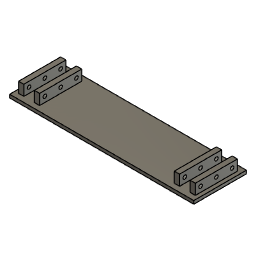
Base v1 (Autodesk Fusion 360 design; units mm, degrees)
Autodesk Fusion 360 part; units mm, degrees
sketch "Sketch1" plane through (0, 0, 0) normal (0, 1, 0) x (1, 0, 0)
  line L0 (-25, 5) -> (150, 5)
  line L1 (150, 5) -> (150, -45)
  line L2 (150, -45) -> (-25, -45)
  line L3 (-25, -45) -> (-25, 5)
  dimension "d1" = 50
  dimension "d2" = 175
  constraint horizontal L0
  constraint vertical L1
  constraint horizontal L2
  constraint vertical L3
  measures "d1" distance of L0.start L2.end
  measures "d2" distance of L0.start L0.end
extrude "Extrude1" add sketch "Sketch1" along normal blind 3
sketch "Sketch2" plane through (0, 3, 0) normal (0, 1, 0) x (-1, 0, 0)
  line L0 (25, 45) -> (-150, 45)
  line L1 (-150, 45) -> (-150, -5)
  line L2 (-150, -5) -> (25, -5)
  line L3 (25, -5) -> (25, 45)
  line L4 (21.5, 0) -> (16.5, 0)
  line L5 (16.5, 0) -> (16.5, 40)
  line L6 (16.5, 40) -> (21.5, 40)
  line L7 (21.5, 40) -> (21.5, 0)
  line L8 (-141.5, 0) -> (-146.5, 0)
  line L9 (-146.5, 0) -> (-146.5, 40)
  line L10 (-146.5, 40) -> (-141.5, 40)
  line L11 (-141.5, 40) -> (-141.5, 0)
  line L12 (6.5, 0) -> (1.5, 0)
  line L13 (1.5, 0) -> (1.5, 40)
  line L14 (1.5, 40) -> (6.5, 40)
  line L15 (6.5, 40) -> (6.5, 0)
  line L16 (-126.5, 0) -> (-131.5, 0)
  line L17 (-131.5, 0) -> (-131.5, 40)
  line L18 (-131.5, 40) -> (-126.5, 40)
  line L19 (-126.5, 40) -> (-126.5, 0)
  dimension "d5" = 158
  dimension "d6" = 5
  dimension "d7" = 40
  dimension "d8" = 40
  dimension "d9" = 5
  dimension "d10" = 3.5
  dimension "d11" = 5
  dimension "d14" = 10
  dimension "d15" = 10
  constraint horizontal L4
  constraint vertical L5
  constraint horizontal L6
  constraint vertical L7
  constraint horizontal L8
  constraint vertical L9
  constraint horizontal L10
  constraint vertical L11
  constraint collinear L6 L10
  constraint horizontal L12
  constraint vertical L13
  constraint horizontal L14
  constraint vertical L15
  constraint horizontal L16
  constraint vertical L17
  constraint horizontal L18
  constraint vertical L19
  constraint collinear L14 L18
  constraint collinear L6 L14
  constraint equal L5 L13
  constraint equal L11 L19
  constraint equal L4 L12
  constraint equal L8 L16
  measures "d5" distance of L5 L11
  measures "d6" distance of L5.end L6.end
  measures "d7" distance of L4.end L5.end
  measures "d8" distance of L8.start L10.end
  measures "d9" distance of L8.start L8.end
  measures "d10" distance of L1 L9
  measures "d11" distance of L0 L6
  measures "d14" distance of L11 L17
  measures "d15" distance of L5 L15
extrude "Extrude2" add sketch "Sketch2" along normal blind 10 contours L4 L5 L6 L7 | L8 L9 L10 L11 | L12 L13 L14 L15 | L16 L17 L18 L19
sketch "Sketch3" plane through (-21.5, 0, 0) normal (-1, 0, 0) x (0, 0, 1)
  line L0 (0, 3) -> (40, 3)
  line L1 (40, 3) -> (40, 13)
  line L2 (40, 13) -> (0, 13)
  line L3 (0, 13) -> (0, 3)
  circle A0 centre (20, 8.1) radius 1.7
  circle A1 centre (35, 8.1) radius 1.7
  circle A2 centre (5, 8.1) radius 1.7
  line L4 (20, 13) -> (20, 3) construction
  dimension "d16" = 3.4
  dimension "d17" = 3.4
  dimension "d18" = 3.4
  dimension "d19" = 15
  dimension "d20" = 15
  dimension "d23" = 5.1
  constraint midpoint L2 L4.start
  constraint midpoint L0 L4.end
  measures "d16" diameter of A2
  measures "d17" diameter of A0
  measures "d18" diameter of A1
  measures "d19" distance of A0.centre A2.centre
  measures "d20" distance of A0.centre A1.centre
  measures "d23" distance of L0 A0.centre
extrude "Extrude3" cut sketch "Sketch3" against normal blind 250 contours A0 | A1 | A2
move_body "Move1" bodies 1 to x (1, 0, 0) y (0, 1, 0) z (0, 0, 1) at (0, 0, 15)
sketch "Sketch4" plane through (0, 0, 0) normal (0, 0, 1) x (1, 0, 0)
